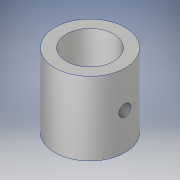
# Autodesk Inventor part: Axle Retainer
Saved by Autodesk Inventor 2019.4 (Build 234330000, 330)
## iProperties
Created: 2019-12-08
Part Number: Axle Retainer
Material: Aluminum 6061
Document SubType Name: Modeling
Designer: admin
Density: 2.7 g/cm^3
Appearance: Aluminum - Flat
Author: admin
Autodesk Inventor part; units mm, degrees
ref_plane "YZ Plane" through (0, 0, 0) normal (1, 0, 0) x (0, 1, 0)
ref_plane "XZ Plane" through (0, 0, 0) normal (0, 1, 0) x (-1, 0, 0)
ref_plane "XY Plane" through (0, 0, 0) normal (0, 0, 1) x (1, 0, 0)
sketch "Sketch1" plane through (0, 0, 0) normal (0, 1, 0) x (-1, 0, 0)
  circle A0 centre (0, 0) radius 10.1
  circle A1 centre (0, 0) radius 15
  dimension "d0" = 20.2
  dimension "d1" = 30
  constraints: 2 centre point, 2 coincident
  measures "d0" diameter of A0
  measures "d1" diameter of A1
extrude "Extrusion1" add sketch "Sketch1" along normal blind 31.3
sketch "Sketch2" plane through (0, 0, 0) normal (1, 0, 0) x (0, 1, 0)
  circle A0 centre (15.65, 0) radius 2.5
  line L0 (15.65, 0) -> (15.65, -15) construction
  line L1 (0, -15) -> (31.3, -15) projected
  point P0 (0, 0)
  dimension "d4" = 5
  constraints: 2 end point, 1 centre point, 1 midpoint, 1 vertical
  measures "d4" diameter of A0
extrude "Extrusion2" cut sketch "Sketch2" along normal through all both and the other way through all
thread "Thread1" size "M5x0.8" class "6H" standard "ANSI Metric M Profile" full length
thread "Thread2" size "M5x0.8" class "6H" standard "ANSI Metric M Profile" full length
body "Solid1"
